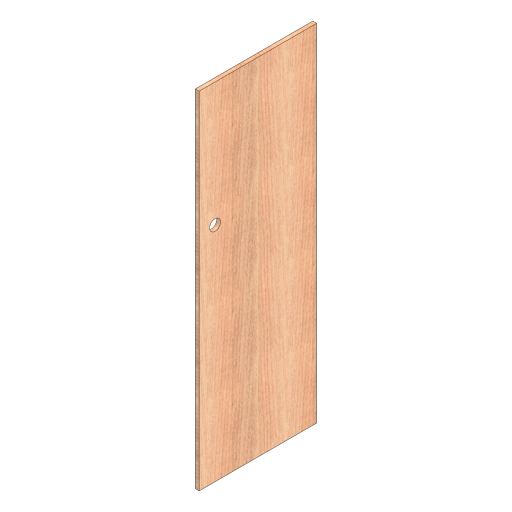
# Autodesk Inventor part: CUT PART R-01
Saved by Autodesk Inventor 2023.2 (Build 272271000, 271)
## iProperties
Created: 2022-12-01
Part Number: CUT PART R-01
Material: Wood (Birch)
Document SubType Name: Modeling
Designer: GUT
Mass: 2442 g
Surface Area: 7728.8 cm^2
Volume: 4440 cm^3
Density: 0.55 g/cm^3
Appearance: Birch - Natural Polished
Author: GUT
Autodesk Inventor part; units mm, degrees
ref_plane "YZ Plane" through (0, 0, 0) normal (1, 0, 0) x (0, 1, 0)
ref_plane "XZ Plane" through (0, 0, 0) normal (0, 1, 0) x (-1, 0, 0)
ref_plane "XY Plane" through (0, 0, 0) normal (0, 0, 1) x (1, 0, 0)
sketch "Sketch1" plane through (0, 0, 0) normal (1, 0, 0) x (0, 1, 0)
  line L0 (-756.0177, 341.6224) -> (333.9823, 341.6224)
  line L1 (333.9823, 341.6224) -> (333.9823, -28.3776)
  line L2 (333.9823, -28.3776) -> (-756.0177, -28.3776)
  line L3 (-756.0177, -28.3776) -> (-756.0177, 341.6224)
  point P0 (0, 0)
  dimension "d0" = 370
  dimension "d1" = 1090
  constraints: 8 end point, 2 parallel, 1 horizontal, 1 perpendicular
  measures "d0" distance of L0.end L1.end
  measures "d1" distance of L0.start L0.end
extrude "Extrusion1" add sketch "Sketch1" along normal blind 12
sketch "Sketch2" plane through (12, 0, 0) normal (1, 0, 0) x (0, 0, -1)
  line L0 (28.3776, -756.0177) -> (28.3776, 333.9823) projected
  line L1 (28.3776, 333.9823) -> (-341.6224, 333.9823) projected
  line L2 (-341.6224, 333.9823) -> (-341.6224, -756.0177) projected
  line L3 (-341.6224, -756.0177) -> (28.3776, -756.0177) projected
  circle A0 centre (-291.6224, -56.0177) radius 17.5
  dimension "d4" = 35
  dimension "d5" = 50
  dimension "d6" = 700
  constraints: 1 centre point
  measures "d4" diameter of A0
  measures "d5" distance from line of L2 A0.centre
  measures "d6" distance from line of L3 A0.centre
extrude "Extrusion2" cut sketch "Sketch2" against normal up to next contours A0
body "Solid1"
